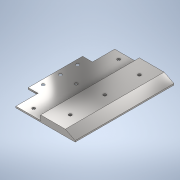
# Autodesk Inventor part: Base Aço
Saved by Autodesk Inventor 2021 (Build 250183000, 183)
## iProperties
Created: 2022-10-28
Part Number: Base Aço
Material: Aço
Document SubType Name: Modeling
Designer: nicho
Density: 7.85 g/cm^3
Appearance: Aço - Polido
Mass: 179.41 g
Surface Area: 144.269 cm^2
Volume: 22.8547 cm^3
Author: nicho
Autodesk Inventor part; units mm, degrees
ref_plane "YZ Plane" through (0, 0, 0) normal (1, 0, 0) x (0, 1, 0)
ref_plane "XZ Plane" through (0, 0, 0) normal (0, 1, 0) x (-1, 0, 0)
ref_plane "XY Plane" through (0, 0, 0) normal (0, 0, 1) x (1, 0, 0)
sketch "Esboço1" plane through (0, 0, 0) normal (0, 1, 0) x (-1, 0, 0)
  line L0 (-35, -50) -> (35, -50)
  line L1 (35, -50) -> (35, 50)
  line L2 (35, 50) -> (-35, 50)
  line L3 (-35, 50) -> (-35, -50)
  line L4 (-35, -50) -> (35, 50) construction
  line L5 (35, -50) -> (-35, 50) construction
  point P0 (0, 0)
  dimension "d0" = 70
  dimension "d1" = 100
  constraints: 12 end point, 2 midpoint, 2 parallel, 1 horizontal, 1 perpendicular
  measures "d0" distance of L2.end L1.end
  measures "d1" distance of L1.end L0.end
extrude "Extrusão1" add sketch "Esboço1" along normal blind 6.35
sketch "Esboço2" plane through (35, 0, -50) normal (0, 0, -1) x (-1, 0, 0)
  line L0 (10, 6.35) -> (0, 1.3533)
  line L1 (0, 1.3533) -> (37.5, 1.3533) construction
  line L2 (0, 0) -> (0, 6.35) projected
  line L3 (0, 6.35) -> (70, 6.35) projected
  line L4 (0, 0) -> (70, 0) projected
  line L5 (70, 0) -> (70, 6.35) projected
  line L6 (0, 6.35) -> (70, 6.35) projected
  line L7 (0, 0) -> (0, 6.35) projected
  line L8 (10, 6.35) -> (35, 6.35)
  line L9 (70, 6.35) -> (0, 6.35) projected
  line L10 (35, 6.35) -> (35, 1.5)
  line L11 (35, 1.5) -> (70, 1.5)
  line L12 (70, 0) -> (70, 6.35) projected
  point P0 (35, 0)
  point P1 (70, 1.5)
  point P2 (35, 6.35)
  dimension "d7" = 25
  dimension "d8" = 26.55
  dimension "d9" = 1.5
  dimension "d16" = 35
  constraints: 10 end point, 3 point on line, 2 horizontal, 1 midpoint, 1 vertical
  measures "d7" distance of L0.start L8.end
  measures "d8" angle of L1 L0
  measures "d9" distance from line of L4 L10.end
  measures "d16" distance of L10.end L11.end
extrude "Extrusão2" cut sketch "Esboço2" against normal through all contours L0 L2 L3 | L3 L5 L11 L10
sketch "Esboço3" plane through (-35, 1.5, -50) normal (0, 1, 0) x (1, 0, 0)
  line L0 (0, -77.5) -> (10, -77.5)
  line L1 (10, -77.5) -> (10, -22.5)
  line L2 (10, -22.5) -> (0, -22.5)
  line L3 (0, -22.5) -> (0, -77.5)
  line L4 (0, -77.5) -> (10, -22.5) construction
  line L5 (10, -77.5) -> (0, -22.5) construction
  line L6 (0, -100) -> (0, 0) projected
  line L7 (35, -100) -> (0, -100) projected
  line L8 (35, 0) -> (35, -100) projected
  line L9 (0, 0) -> (35, 0) projected
  line L10 (0, -100) -> (0, 0) projected
  line L11 (10, -77.5) -> (10, -100)
  line L12 (0, -100) -> (70, -100) projected
  line L13 (10, -22.5) -> (10, 0)
  line L14 (70, 0) -> (0, 0) projected
  point P0 (35, -50)
  point P1 (5, -50)
  point P2 (5, -50)
  point P3 (10, -100)
  dimension "d12" = 10
  dimension "d13" = 55
  constraints: 16 end point, 4 point on line, 3 midpoint, 2 parallel, 1 horizontal, 1 horizontal alignment, 1 perpendicular, 1 vertical
  measures "d12" distance of L2.end L1.end
  measures "d13" distance of L1.end L0.end
extrude "Extrusão3" cut sketch "Esboço3" against normal through all contours L0 L11 L7 L6 | L6 L9 L13 L2
sketch "Esboço10" plane through (0, 1.5, 50) normal (0, 1, 0) x (1, 0, 0)
  line L0 (-35, 22.5) -> (-25, 22.5) projected
  line L1 (-25, 77.5) -> (-35, 77.5) projected
  line L2 (0, 0) -> (-25, 0) projected
  line L3 (-25, 22.5) -> (-25, 0) projected
  point P0 (0, 50)
  point P1 (-30, 32.5)
  point P2 (-30, 50)
  point P3 (-30, 67.5)
  dimension "d61" = 10
  dimension "d62" = 10
  dimension "d63" = 50
  dimension "d64" = 5
  constraints: 2 vertical alignment
  measures "d61" distance from line of L0 point (-30, 32.5)
  measures "d62" distance from line of L1 point (-30, 67.5)
  measures "d63" distance from line of L2 point (-30, 50)
  measures "d64" distance from line of L3 point (-30, 32.5)
hole "Furo3" at (-30, 1.5, 17.5) at (-30, 1.5, 0) at (-30, 1.5, -17.5) direction (0, -1, 0) diameter 3 end through all
chamfer "Chanfro1" distance 1.5 angle 45 3 edges at (-30, 0, -19) (-30, 0, -1.5) (-30, 0, 16)
sketch "Esboço11" plane through (0, 6.35, 0) normal (0, 1, 0) x (1, 0, 0)
  line L0 (0, 50) -> (0, -50) projected
  line L1 (25, -50) -> (25, 50) projected
  point P0 (0, 0)
  point P1 (15, -35)
  point P2 (15, 0)
  point P3 (15, 35)
  point P4 (0, 0)
  point P5 (-14, 0)
  point P6 (-14, -43)
  point P7 (-14, 43)
  dimension "d75" = 10
  dimension "d76" = 35
  dimension "d77" = 35
  dimension "d78" = 29
  dimension "d79" = 43
  dimension "d80" = 43
  constraints: 4 vertical alignment, 2 horizontal alignment, 1 midpoint
  measures "d75" distance from line of L1 point (15, 0)
  measures "d76" distance of point (15, 0) point (15, -35)
  measures "d77" distance of point (15, 35) point (15, 0)
  measures "d78" distance of point (15, 0) point (-14, 0)
  measures "d79" vertical distance of point (15, 0) point (-14, -43)
  measures "d80" distance of point (-14, 43) point (-14, 0)
hole "Furo4" at (15, 6.35, 35) at (15, 6.35, 0) at (15, 6.35, -35) at (-14, 6.35, 0) at (-14, 6.35, 43) at (-14, 6.35, -43) direction (0, -1, 0) diameter 3 end through all
equation "\"d62\" = d61"
equation "\"d77\" = d76"
equation "\"d80\" = d79"
